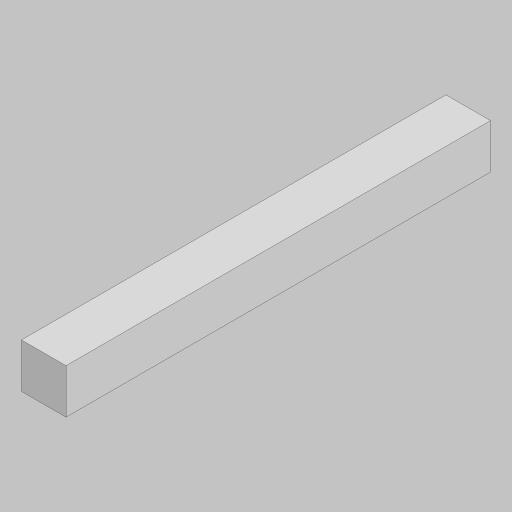
# Autodesk Inventor part: Pines_parametrizado
Saved by Autodesk Inventor 2023 (Build 270158000, 158)
## iProperties
Created: 2026-03-03
Part Number: Pines_parametrizado
Material: Genérico
Document SubType Name: Modeling
Designer: MARTIN MAESTRE
Density: 1 g/cm^3
Appearance: Valor por defecto
Author: MARTIN MAESTRE
Autodesk Inventor part; units mm, degrees
ref_plane "YZ Plane" through (0, 0, 0) normal (1, 0, 0) x (0, 1, 0)
ref_plane "XZ Plane" through (0, 0, 0) normal (0, 1, 0) x (-1, 0, 0)
ref_plane "XY Plane" through (0, 0, 0) normal (0, 0, 1) x (1, 0, 0)
sketch "Boceto1" plane through (0, 0, 0) normal (0, 0, 1) x (1, 0, 0)
  line L0 (0, 0) -> (4.2, 0)
  line L1 (4.2, 0) -> (4.2, 4.2)
  line L2 (4.2, 4.2) -> (0, 4.2)
  line L3 (0, 4.2) -> (0, 0)
  dimension "d0" = 4.2
  dimension "d1" = 4.2
  constraints: 8 end point, 2 parallel, 1 horizontal, 1 perpendicular
  measures "d0" distance of L2.end L1.end
  measures "d1" distance of L1.end L0.end
extrude "Extrusión1" add sketch "Boceto1" along normal blind 40
equation "\"d0\" = Ancho"
equation "\"d1\" = Largo"
equation "\"d2\" = Alto"
equation "\"Ancho\" = 4.2 * Escala"
equation "\"Largo\" = 4.2 * Escala"
equation "\"Alto\" = 40 * Escala"
equation "\"Escala\" = 1"
